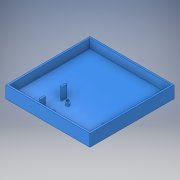
# Autodesk Inventor part: LargeCaseBottomForPiZeroW
Saved by Autodesk Inventor 2019.3 (Build 233278000, 278)
## iProperties
Created: 2018-12-18
Part Number: LargeCaseBottomForPiZeroW
Material: LCP Plastic
Document SubType Name: Modeling
Designer: steele
Density: 1.626 g/cm^3
Appearance: Cyan
PiZeroWLength: 2.559 in
PiZeroWWidth: 1.181 in
CaseLength: 3.150 in
CaseWidth: 1.772 in
CaseHeight: 0.515 in
PiZeroWMountingHole: 0.108 in
CaseWallThickness: 0.100 in
CaseFloorThickness: 0.200 in
PiZeroMoutingHolesLength: 2.283 in
PiZeroMountingHolesWidth: 0.906 in
PiZeroHoleSupport: 0.236 in
PiZeroWHoleHeight: 0.100 in
PiRibbonCableWidth: 0.787 in
PiRibbonCableThickness: 0.197 in
HdmiCenter: 0.748 in
MiniUsbCenter: 1.630 in
PowerCenter: 2.126 in
HdmiWidth: 1.102 in
MiniUsbWidth: 0.709 in
PowerWidth: 0.787 in
EndOfCaseToStartOfPiZero: 0.295 in
EyepieceOutsideDiameter: 1.250 in
EyepieceWallThickness: 0.075 in
EyepieceInnerDiameter: 1.100 in
PiRibbonCableHeightFromTp: 0.350 in
NutHeightPlusOffset: 0.073 in
NutWidthPlusOffset: 0.198 in
FilletForRibbonCable: 0.033 in
Author: steele
Autodesk Inventor part; units mm, degrees
ref_plane "YZ Plane" through (0, 0, 0) normal (1, 0, 0) x (0, 1, 0)
ref_plane "XZ Plane" through (0, 0, 0) normal (0, 1, 0) x (-1, 0, 0)
ref_plane "XY Plane" through (0, 0, 0) normal (0, 0, 1) x (1, 0, 0)
sketch "Sketch1" plane through (0, 0, 0) normal (0, 1, 0) x (-1, 0, 0)
  line L0 (38.73, 21.23) -> (-38.73, 21.23)
  line L1 (-38.73, 21.23) -> (-38.73, -21.23)
  line L2 (-38.73, -21.23) -> (38.73, -21.23)
  line L3 (38.73, -21.23) -> (38.73, 21.23)
  line L4 (38.73, 21.23) -> (-38.73, -21.23) construction
  line L5 (-38.73, 21.23) -> (38.73, -21.23) construction
  line L6 (38.73, -21.23) -> (-38.73, -21.23)
  line L7 (-38.73, -21.23) -> (-38.73, -105.77)
  line L8 (-38.73, -105.77) -> (38.73, -105.77)
  line L9 (38.73, -105.77) -> (38.73, -21.23)
  line L10 (38.73, -105.77) -> (88.27, -105.77)
  line L11 (88.27, -105.77) -> (88.27, 21.23)
  line L12 (88.27, 21.23) -> (38.73, 21.23)
  line L13 (38.73, 21.23) -> (38.73, -105.77)
  point P0 (0, 0)
  dimension "d0" = 77.46
  dimension "d1" = 42.46
  dimension "overallWidthOfBottom" = 127
  dimension "overallLengthOfBottom" = 127
  constraints: 28 end point, 6 parallel, 3 horizontal, 3 perpendicular, 2 collinear, 2 midpoint
  measures "d0" distance of L1.end L2.end
  measures "d1" distance of L2.end L0.start
  measures "overallWidthOfBottom" distance between parallel lines of L0 L8
  measures "overallLengthOfBottom" distance between parallel lines of L1 L11
extrude "Extrusion1" add sketch "Sketch1" against normal blind 5.08
sketch "Sketch3" plane through (0, 0, 0) normal (0, 1, 0) x (1, 0, 0)
  line L0 (-29, -11.5) -> (29, -11.5) construction
  line L1 (29, -11.5) -> (29, 11.5) construction
  line L2 (29, 11.5) -> (-29, 11.5) construction
  line L3 (-29, 11.5) -> (-29, -11.5) construction
  line L4 (-29, -11.5) -> (29, 11.5) construction
  line L5 (29, -11.5) -> (-29, 11.5) construction
  circle A0 centre (-29, -11.5) radius 3
  circle A1 centre (29, -11.5) radius 3
  circle A2 centre (-29, 11.5) radius 3
  circle A3 centre (29, 11.5) radius 3
  point P0 (0, 0)
  dimension "d8" = 23
  dimension "d9" = 58
  dimension "d19" = 58
  dimension "d22" = 23
  dimension "d25" = 6
  constraints: 12 end point, 4 centre point, 2 coincident, 2 horizontal, 2 midpoint, 2 parallel, 1 perpendicular, 1 vertical, 6 other
  measures "d8" distance of L2.end L0.start
  measures "d9" distance of L1.end L2.end
  measures "d19" distance of A0.centre A1.centre
  measures "d22" distance of A0.centre A2.centre
  measures "d25" diameter of A0
extrude "Extrusion3" add sketch "Sketch3" along normal blind 2.54
sketch "Sketch22" plane through (0, -5.08, 0) normal (0, -1, 0) x (1, 0, 0)
  point P0 (34.92, -17.42)
  point P1 (34.92, 17.42)
  point P2 (-34.92, 17.42)
  point P3 (-34.92, -17.42)
hole "Hole12" at (34.92, -5.08, -17.42) at (34.92, -5.08, 17.42) at (-34.92, -5.08, 17.42) at (-34.92, -5.08, -17.42) direction (0, 1, 0) diameter 3.7973 depth 5.08
sketch "Sketch23" plane through (0, -5.08, 0) normal (0, -1, 0) x (1, 0, 0)
  circle A0 centre (-34.92, 17.42) radius 1.8986 projected
  circle A1 centre (34.92, 17.42) radius 1.8986 projected
  circle A2 centre (34.92, -17.42) radius 1.8986 projected
  circle A3 centre (-34.92, -17.42) radius 1.8986 projected
  point P0 (0, 0)
  constraints: 4 coincident
hole "Hole13" at (-34.92, -5.08, 17.42) at (34.92, -5.08, 17.42) at (34.92, -5.08, -17.42) at (-34.92, -5.08, -17.42) direction (0, 1, 0) diameter 4.8514 depth 3.81
sketch "Sketch25" plane through (0, -5.08, 0) normal (0, -1, 0) x (1, 0, 0)
  circle A0 centre (29, 11.5) radius 3 projected
  circle A1 centre (29, -11.5) radius 3 projected
  circle A2 centre (-29, -11.5) radius 3 projected
  circle A3 centre (-29, 11.5) radius 3 projected
  point P0 (0, 0)
  constraints: 4 coincident
hole "Hole16" at (29, -5.08, 11.5) at (29, -5.08, -11.5) at (-29, -5.08, -11.5) at (-29, -5.08, 11.5) direction (0, 1, 0) diameter 2.4384 end through all counterbore diameter 3.2639 counterbore depth 3.9878
sketch "Sketch26" plane through (0, -5.08, 0) normal (0, -1, 0) x (1, 0, 0)
  line L0 (-88.27, -105.77) -> (38.73, -105.77) projected
  line L1 (-88.27, 21.23) -> (38.73, 21.23)
  line L2 (38.73, 21.23) -> (38.73, -105.77)
  line L3 (38.73, -105.77) -> (-88.27, -105.77)
  line L4 (-88.27, -105.77) -> (-88.27, 21.23)
  line L5 (-90.81, 23.77) -> (41.27, 23.77)
  line L6 (41.27, 23.77) -> (41.27, -108.31)
  line L7 (41.27, -108.31) -> (-90.81, -108.31)
  line L8 (-90.81, -108.31) -> (-90.81, 23.77)
  point P0 (0, 0)
  dimension "d175" = 2.54
  dimension "d176" = 2.54
  dimension "d177" = 2.54
  dimension "d178" = 2.54
  constraints: 16 end point, 4 parallel, 2 horizontal, 2 perpendicular
  measures "d175" distance between parallel lines of L1 L5
  measures "d176" distance between parallel lines of L0 L7
  measures "d177" distance between parallel lines of L8 L4
  measures "d178" distance between parallel lines of L2 L6
extrude "Extrusion12" add sketch "Sketch26" against normal blind 19.05
sketch "Sketch27" plane through (0, 0, 0) normal (0, 1, 0) x (1, 0, 0)
  line L0 (-88.27, -21.23) -> (38.73, -21.23) projected
  line L1 (-38.74, -21.23) -> (-41.28, -21.23)
  line L2 (-41.28, -21.23) -> (-41.28, -13.61)
  line L3 (-41.28, -13.61) -> (-38.74, -13.61)
  line L4 (-38.74, -13.61) -> (-38.74, -21.23)
  line L5 (-38.74, 11.79) -> (-41.28, 11.79)
  line L6 (-41.28, 11.79) -> (-41.28, 19.918)
  line L7 (-41.28, 19.918) -> (-38.74, 19.918)
  line L8 (-38.74, 19.918) -> (-38.74, 11.79)
  line L9 (38.73, 105.77) -> (38.73, -21.23) projected
  circle A0 centre (34.92, -17.42) radius 1.8986 projected
  point P0 (0, 0)
  dimension "d181" = 77.47
  dimension "d182" = 2.54
  dimension "d183" = 7.62
  dimension "d184" = 3.81
  dimension "d185" = 41.148
  dimension "d186" = 25.4
  constraints: 16 end point, 4 parallel, 2 collinear, 2 horizontal, 2 perpendicular, 1 point on line
  measures "d181" distance between parallel lines of L9 L4
  measures "d182" distance between parallel lines of L2 L4
  measures "d183" distance of L1.end L2.end
  measures "d184" distance from line of L0 A0.centre
  measures "d185" distance between parallel lines of L7 L0
  measures "d186" distance between parallel lines of L5 L3
extrude "Extrusion13" add sketch "Sketch27" along normal blind 19.05 contours L2 L3 L4 L0 | L5 L6 L7 L8
equation "\"d2\" = CaseFloorThickness"
equation "\"d8\" = PiZeroMountingHolesWidth"
equation "\"d9\" = PiZeroMoutingHolesLength"
equation "\"d19\" = PiZeroMoutingHolesLength"
equation "\"d22\" = PiZeroMountingHolesWidth"
equation "\"d25\" = PiZeroHoleSupport"
equation "\"d26\" = PiZeroWHoleHeight"
equation "\"d175\" = CaseWallThickness"
equation "\"d176\" = CaseWallThickness"
equation "\"d177\" = CaseWallThickness"
equation "\"d178\" = CaseWallThickness"
equation "\"PiZeroWLength\" = 65"
equation "\"PiZeroWWidth\" = 30"
equation "\"CaseLength\" = PiZeroWLength + 2 * EndOfCaseToStartOfPiZero"
equation "\"CaseWidth\" = PiZeroWWidth + 2 * EndOfCaseToStartOfPiZero"
equation "\"PiZeroWMountingHole\" = 2.75"
equation "\"CaseWallThickness\" = 2.54"
equation "\"CaseFloorThickness\" = 5.08"
equation "\"PiZeroMoutingHolesLength\" = 58"
equation "\"PiZeroMountingHolesWidth\" = 23"
equation "\"PiZeroHoleSupport\" = 6"
equation "\"PiZeroWHoleHeight\" = 2.54"
equation "\"PiRibbonCableWidth\" = 20"
equation "\"PiRibbonCableThickness\" = 5"
equation "\"HdmiCenter\" = 19"
equation "\"MiniUsbCenter\" = 41.4"
equation "\"PowerCenter\" = 54"
equation "\"HdmiWidth\" = 28"
equation "\"MiniUsbWidth\" = 18"
equation "\"PowerWidth\" = 20"
equation "\"EndOfCaseToStartOfPiZero\" = 7.5"
equation "\"EyepieceOutsideDiameter\" = 31.75"
equation "\"EyepieceWallThickness\" = 1.905"
equation "\"EyepieceInnerDiameter\" = EyepieceOutsideDiameter - 2 * EyepieceWallThickness"
equation "\"HeightOfConnectorHolesAboveBottom\" = 6"
equation "\"HdmiHightAboveBottom\" = 6"
equation "\"MiniUsbHeightAboveBottom\" = 5"
equation "\"PowerHeightAboveBottom\" = 5"
equation "\"PiRibbonCableHeightFromTp\" = 8.89"
equation "\"NutHeightPlusOffset\" = 1.8415"
equation "\"NutWidthPlusOffset\" = 5.0165"
equation "\"FilletForRibbonCable\" = 0.333333 * CaseWallThickness"
body "Solid1"
